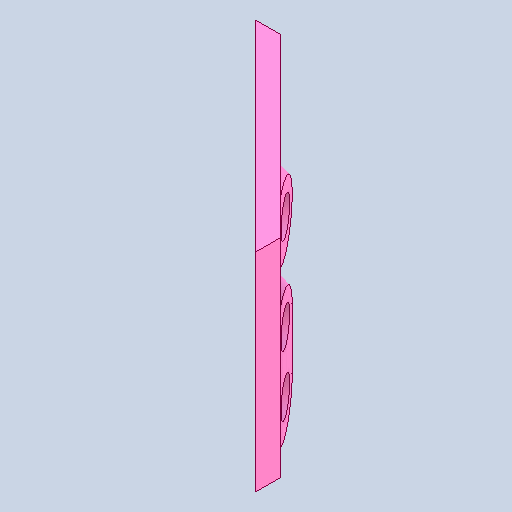
# Autodesk Inventor part: Mirror Plate
Saved by Autodesk Inventor 2023.1 (Build 271208000, 208)
## iProperties
Created: 2022-08-09
Part Number: Mirror Plate
Material: Generic
Document SubType Name: Modeling
Designer: xSibe
Density: 1 g/cm^3
Appearance: Plastic Pink
Author: xSibe
Autodesk Inventor part; units mm, degrees
ref_plane "YZ Plane" through (0, 0, 0) normal (1, 0, 0) x (0, 1, 0)
ref_plane "Work Plane1" through (-24.9, -24.9, 7.7) normal (0, 0, 1) x (1, 0, 0)
sketch "Sketch1" plane through (0, 0, 0) normal (0, 0, 1) x (0, 1, 0)
  circle A0 centre (20.9, 10) radius 1.875 projected
  circle A1 centre (-20.9, 10) radius 1.875 projected
  circle A2 centre (20.9, -10) radius 1.875 projected
  circle A3 centre (-20.9, -10) radius 1.875 projected
  circle A4 centre (-14.4, -20.8) radius 2.0675 projected
  circle A5 centre (14.4, -20.8) radius 2.0675 projected
  circle A6 centre (14.4, 20.8) radius 2.0675 projected
  circle A7 centre (-14.4, 20.8) radius 2.0675 projected
  line L0 (-16.9, -16.9) -> (-16.9, 16.9) projected
  line L1 (-16.9, 16.9) -> (16.9, 16.9) projected
  line L2 (16.9, 16.9) -> (16.9, -16.9) projected
  line L3 (16.9, -16.9) -> (-16.9, -16.9) projected
  line L4 (24.9, 17.05) -> (22.55, 17.05) projected
  line L5 (22.55, 17.05) -> (17.05, 22.55) projected
  line L6 (17.05, 22.55) -> (17.05, 24.9) projected
  line L7 (17.05, 24.9) -> (-17.05, 24.9) projected
  line L8 (-17.05, 24.9) -> (-17.05, 22.55) projected
  line L9 (-17.05, 22.55) -> (-22.55, 17.05) projected
  line L10 (-22.55, 17.05) -> (-24.9, 17.05) projected
  line L11 (-24.9, 17.05) -> (-24.9, -17.05) projected
  line L12 (-24.9, -17.05) -> (-22.55, -17.05) projected
  line L13 (-22.55, -17.05) -> (-17.05, -22.55) projected
  line L14 (-17.05, -22.55) -> (-17.05, -24.9) projected
  line L15 (-17.05, -24.9) -> (17.05, -24.9) projected
  line L16 (17.05, -24.9) -> (17.05, -22.55) projected
  line L17 (17.05, -22.55) -> (22.55, -17.05) projected
  line L18 (22.55, -17.05) -> (24.9, -17.05) projected
  line L19 (24.9, -17.05) -> (24.9, 17.05) projected
  line L20 (16.975, -24.825) -> (-16.975, -24.825)
  line L21 (-16.975, -24.825) -> (-16.975, -22.5189)
  line L22 (-16.975, -22.5189) -> (-22.5189, -16.975)
  line L23 (-22.5189, -16.975) -> (-24.825, -16.975)
  line L24 (-24.825, -16.975) -> (-24.825, 16.975)
  line L25 (-24.825, 16.975) -> (-22.5189, 16.975)
  line L26 (-22.5189, 16.975) -> (-16.975, 22.5189)
  line L27 (-16.975, 22.5189) -> (-16.975, 24.825)
  line L28 (-16.975, 24.825) -> (16.975, 24.825)
  line L29 (16.975, 24.825) -> (16.975, 22.5189)
  line L30 (16.975, 22.5189) -> (22.5189, 16.975)
  line L31 (22.5189, 16.975) -> (24.825, 16.975)
  line L32 (24.825, 16.975) -> (24.825, -16.975)
  line L33 (24.825, -16.975) -> (22.5189, -16.975)
  line L34 (22.5189, -16.975) -> (16.975, -22.5189)
  line L35 (16.975, -22.5189) -> (16.975, -24.825)
  dimension "d5" = 0.075
  constraints: 32 end point, 15 other
  measures "d5" distance between parallel lines of L15 L20
extrude "Extrusion1" add sketch "Sketch1" along normal blind 2.5 from surface at 7.7 contours A0 | A1 | A2 | A3 | A4 | A5 | A6 | A7 | L0 L1 L2 L3 | L20 L21 L22 L23 L24 L25 L26 L27 L28 L29 L30 L31 L32 L33 L34 L35
sketch "Sketch2" plane through (0, 0, 0) normal (0, 1, 0) x (-1, 0, 0)
  line L0 (16.975, 10.2) -> (-16.975, 10.2) projected
  line L1 (-16.975, 7.7) -> (-16.975, 10.2) projected
  line L2 (16.975, 7.7) -> (-16.975, 7.7) projected
  line L3 (16.975, 7.7) -> (16.975, 10.2) projected
  line L4 (16.975, 7.7) -> (-16.975, 41.65)
  line L5 (16.975, 7.7) -> (64.9876, 7.7) construction
  line L6 (-16.975, 41.65) -> (-16.975, 10.2)
  line L7 (-20.5105, 41.65) -> (10.9395, 10.2)
  line L8 (7.4039, 10.2) -> (-24.0461, 41.65)
  line L9 (-19.475, 12.7) -> (19.475, 12.7)
  line L10 (19.475, 12.7) -> (19.475, 5.2)
  line L11 (19.475, 5.2) -> (-19.475, 5.2)
  line L12 (-19.475, 5.2) -> (-19.475, 12.7)
  line L13 (-16.975, 41.65) -> (-24.825, 41.65)
  line L14 (-24.825, 41.65) -> (-24.825, 10.2)
  line L15 (-24.825, 10.2) -> (-16.975, 10.2)
  line L16 (-16.975, 10.2) -> (-16.975, 41.65)
  point P0 (0, 0)
  point P1 (14.475, 10.2)
  point P2 (-16.975, 38.1145)
  point P3 (-16.975, 34.5789)
  point P4 (8.4395, 12.7)
  point P5 (11.975, 12.7)
  point P6 (-19.475, 10.2)
  point P7 (-16.975, 12.7)
  point P8 (-16.975, 10.2)
  dimension "d6" = 135
  dimension "d9" = 2.5
  dimension "d10" = 2.5
  dimension "d13" = 2.5
  constraints: 26 end point, 8 point on line, 2 horizontal, 2 parallel, 2 perpendicular, 1 equal length, 3 other
  measures "d6" angle of L5 L4
  measures "d9" distance between parallel lines of L4 L7
  measures "d10" distance between parallel lines of L7 L8
  measures "d13" distance between parallel lines of L0 L9
extrude "Extrusion2" add sketch "Sketch2" along normal mid plane 30 contours L7 L9 L4 L0 | L0 L8 L9 L7 | L0 L6 L9 L8 | L9 L8 L6 L7 | L7 L6 L4 L9 | L15 L12 L9 L6 | L9 L6 L8 | L7 L13 L6 | L6 L8 L13 L7 | L9 L12 L15 L14 L13 L8 L6
extrude "Extrusion3" cut sketch "Sketch2" along normal mid plane 30 contours L7 L9 L4 L0 | L0 L8 L9 L7 | L9 L8 L6 L7 | L7 L13 L6 | L6 L8 L13 L7
ref_plane "Work Plane2" through (24.825, 0, 41.65) normal (0.9848078, 0, -0.1736482) x (0, 1, 0)
sketch "Sketch3" plane through (20.7643, -15, 18.6207) normal (0.9848078, 0, -0.1736482) x (-0.1736482, 0, -0.9848078)
  line L0 (10.902, 0) -> (-18.5396, 0) projected
  line L1 (10.902, 0) -> (10.902, 30) projected
  line L2 (-18.5396, 30) -> (10.902, 30) projected
  line L3 (-18.5396, 15) -> (10.902, 15)
  line L4 (6.1812, 6.25) -> (-13.8188, 6.25)
  line L5 (-13.8188, 6.25) -> (-13.8188, 23.75)
  line L6 (-13.8188, 23.75) -> (6.1812, 23.75)
  line L7 (6.1812, 23.75) -> (6.1812, 6.25)
  line L8 (6.1812, 6.25) -> (-13.8188, 23.75) construction
  line L9 (-13.8188, 6.25) -> (6.1812, 23.75) construction
  circle A0 centre (-13.8188, 6.25) radius 2.5875
  circle A1 centre (-13.8188, 6.25) radius 5.0875
  line L10 (-3.8188, 15) -> (-3.8188, 6.25)
  line L11 (-3.8188, 10.625) -> (-13.8188, 10.625)
  line L12 (-8.8188, 10.625) -> (-8.8188, 6.25)
  circle A2 centre (-13.8188, 15) radius 2.5875
  circle A3 centre (-13.8188, 15) radius 5.0875
  circle A4 centre (-3.8188, 15) radius 5.0875
  circle A5 centre (-3.8188, 15) radius 2.5875
  line L13 (-18.9063, 6.25) -> (-18.9063, 15)
  line L14 (-8.7313, 15) -> (-8.7313, 6.25)
  line L15 (-18.5396, 0) -> (-18.5396, 30) projected
  point P0 (21.9435, 15)
  dimension "d16" = 20
  dimension "d17" = 17.5
  dimension "d18" = 5.175
  dimension "d19" = 2.5
  constraints: 24 end point, 8 midpoint, 6 centre point, 5 point on line, 4 point on circle, 3 perpendicular, 2 parallel, 1 coincident, 1 horizontal, 1 symmetric about line, 1 tangent, 4 other
  measures "d16" distance of L5.end L6.end
  measures "d17" distance of L4.end L5.end
  measures "d18" diameter of A0
  measures "d19" radial gap between concentric circles of A0 A1
extrude "Extrusion4" cut sketch "Sketch3" along normal mid plane 50 contours A0 L5 L4 | L4 L5 A0 | A2 L3 L5 | L5 L3 A2 | A2 L5 L3 | A2 L3 L5
extrude "Extrusion5" cut sketch "Sketch3" along normal blind 4.25 and the other way blind 2.5 contours L15 A1 A3 L5 A0 L4 | A1 L15 | L13 A3 L15 A1 | L4 L12 A1 | A1 L12 L11 L14 | L15 A3 A1 | A3 L15 | L4 A0 L5 A3 A1 L12 | A1 L11 L12 | L11 A3 A4 L14 | A3 L15 L3 A2 L5 A1 | A1 L5 A3 | A3 L5 A2 L3 L15 | A4 L3 A2 L5 A3 | A3 L3 A4 | A0 L5 L4 | L4 L5 A0 | L11 L5 A1 | A3 L5 L11 | A1 L5 A2 L3 A4 A3 | A4 A3 L14 | A3 A4 L3 | A2 L3 L5 | L5 L3 A2 | A2 L5 L3 | A2 L3 L5
sketch "Sketch4" plane through (17.8921, 0, 2.3313) normal (0.9848078, 0, -0.1736482) x (0, 1, 0)
  line L0 (-15, 5.6387) -> (-15, 35.0803) projected
  line L1 (-15, 5.6387) -> (15, 5.6387) projected
  line L2 (15, 35.0803) -> (15, 5.6387) projected
  circle A0 centre (0, 14.3887) radius 2.5875
  circle A1 centre (0, 14.3887) radius 5.0875
  line L3 (-15, 35.0803) -> (15, 35.0803) projected
  line L4 (0, 5.6387) -> (0, 14.3887)
  point P0 (0, -5.1645)
  dimension "d25" = 5.175
  dimension "d26" = 2.5
  dimension "d37" = 8.75
  constraints: 2 centre point, 2 end point, 1 coincident, 1 midpoint, 1 vertical
  measures "d25" diameter of A0
  measures "d26" radial gap between concentric circles of A0 A1
  measures "d37" distance of L4.start L4.end
extrude "Extrusion6" cut sketch "Sketch4" along normal mid plane 100 contours A0
extrude "Extrusion7" cut sketch "Sketch4" along normal blind 15 and the other way blind 10 contours A0 | A1
sketch "Sketch7" plane through (-3.5875, 0, 17.552) normal (0, 1, 0) x (-0.7071068, 0, -0.7071068)
  line L0 (-20.158, 0) -> (-26.4755, 0) projected
  line L1 (-0.6613, 0) -> (-6.9788, 0) projected
  line L2 (1.0892, 2.5) -> (-0.6613, 0) projected
  line L3 (-5.2283, 2.5) -> (1.0892, 2.5) projected
  line L4 (-5.2283, 2.5) -> (-6.9788, 0) projected
  line L5 (-18.4075, 2.5) -> (-20.158, 0) projected
  line L6 (-24.725, 2.5) -> (-18.4075, 2.5) projected
  line L7 (-24.725, 2.5) -> (-26.4755, 0) projected
  line L8 (-3.8201, 0) -> (-4.0701, 0)
  line L9 (-23.3168, 0) -> (-23.5668, 0)
  line L10 (-1.7448, -1.4254) -> (-6.7427, -0.5442)
  line L11 (-6.7427, -0.5442) -> (-6.3954, 1.4254)
  line L12 (-6.3954, 1.4254) -> (-1.3975, 0.5442)
  line L13 (-1.3975, 0.5442) -> (-1.7448, -1.4254)
  line L14 (-1.7448, -1.4254) -> (-6.3954, 1.4254) construction
  line L15 (-6.7427, -0.5442) -> (-1.3975, 0.5442) construction
  line L16 (-1.7448, -1.4254) -> (3.3302, -1.4254) construction
  line L17 (-21.2415, -1.4254) -> (-26.2394, -0.5442)
  line L18 (-26.2394, -0.5442) -> (-25.8921, 1.4254)
  line L19 (-25.8921, 1.4254) -> (-20.8942, 0.5442)
  line L20 (-20.8942, 0.5442) -> (-21.2415, -1.4254)
  line L21 (-21.2415, -1.4254) -> (-25.8921, 1.4254) construction
  line L22 (-26.2394, -0.5442) -> (-20.8942, 0.5442) construction
  line L23 (-21.2415, -1.4254) -> (-16.1665, -1.4254) construction
  line L24 (-27.1088, 3.1631) -> (-27.9771, -1.7609)
  line L25 (-27.9771, -1.7609) -> (-20.0247, -3.1631)
  line L26 (-20.0247, -3.1631) -> (-19.1565, 1.7609)
  line L27 (-19.1565, 1.7609) -> (-27.1088, 3.1631)
  line L28 (-7.6121, 3.1631) -> (-8.4804, -1.7609)
  line L29 (-8.4804, -1.7609) -> (-0.528, -3.1631)
  line L30 (-0.528, -3.1631) -> (0.3402, 1.7609)
  line L31 (0.3402, 1.7609) -> (-7.6121, 3.1631)
  line L32 (-0.6613, 0) -> (0.0297, 0)
  line L33 (-20.158, 0) -> (-19.467, 0)
  line L34 (-1.7448, -1.4254) -> (0.0297, 0)
  line L35 (-21.2415, -1.4254) -> (-19.467, 0)
  line L36 (-26.4755, 0) -> (-27.6666, 0)
  line L37 (-6.9788, 0) -> (-8.1699, 0)
  line L38 (-6.7427, -0.5442) -> (-8.1699, 0)
  line L39 (-26.2394, -0.5442) -> (-27.6666, 0)
  point P0 (-1.4934, 0)
  point P1 (-6.6467, 0)
  point P2 (-26.1434, 0)
  point P3 (-20.9901, 0)
  dimension "d70" = 0.25
  dimension "d71" = 0.25
  dimension "d72" = 5.075
  dimension "d73" = 170
  dimension "d74" = 2
  dimension "d75" = 5.075
  dimension "d76" = 170
  dimension "d77" = 2
  dimension "d78" = 1.5
  dimension "d79" = 1.5
  constraints: 64 end point, 8 parallel, 8 point on line, 6 midpoint, 5 perpendicular, 4 horizontal, 2 equal length, 6 other
  measures "d70" distance of L8.start L8.end
  measures "d71" distance of L9.start L9.end
  measures "d72" distance of L10.start L10.end
  measures "d73" angle of L16 L10
  measures "d74" distance of L10.end L11.end
  measures "d75" distance of L17.start L17.end
  measures "d76" angle of L23 L17
  measures "d77" distance of L17.end L18.end
  measures "d78" distance between parallel lines of L18 L24
  measures "d79" distance between parallel lines of L11 L28
extrude "Extrusion10" add sketch "Sketch7" along normal mid plane 30 contours L0 L18 L7 L19 L20 | L20 L19 L7 L6 L27 L26 L5 L0 | L0 L7 L18 | L26 L27 L6 L5 | L1 L11 L4 L12 L13 | L13 L12 L4 L3 L31 L30 L2 L1 | L1 L4 L11 | L30 L31 L3 L2
extrude "Extrusion11" cut sketch "Sketch7" along normal mid plane 5.075 contours L0 L20 L17 L18 | L0 L18 L7 L19 L20 | L18 L19 L7 | L1 L13 L10 L11 | L1 L11 L4 L12 L13 | L11 L12 L4
sketch "Sketch8" plane through (13.713, -15.0375, 36.8684) normal (0.819152, 0, -0.5735764) x (-0.5735764, 0, -0.819152)
  line L0 (0, 12.5) -> (0, 17.575) projected
  line L1 (5.075, 17.575) -> (5.075, 12.5) projected
  line L2 (0, 12.5) -> (5.075, 12.5) projected
  line L3 (5.075, 17.575) -> (0, 17.575) projected
  line L4 (2.5375, 12.5) -> (2.5375, 17.575)
  circle A0 centre (2.5375, 15.0375) radius 2.5375
  circle A1 centre (2.5375, 15.0375) radius 4.0375
  circle A2 centre (2.5375, 6.2875) radius 4.0375
  circle A3 centre (2.5375, 6.2875) radius 2.5375
  line L5 (-1.5, 6.2875) -> (-1.5, 15.0375)
  line L6 (6.575, 6.2875) -> (6.575, 15.0375)
  point P0 (38.0663, 15.0375)
  dimension "d86" = 5.075
  dimension "d87" = 1.5
  dimension "d90" = 8.75
  constraints: 6 end point, 4 centre point, 4 point on circle, 4 tangent, 3 midpoint, 1 vertical, 3 other
  measures "d86" diameter of A0
  measures "d87" radial gap between concentric circles of A0 A1
  measures "d90" distance of A0.centre A3.centre
extrude "Extrusion12" cut sketch "Sketch8" along normal blind 1.5 contours A0 L4 | L4 A0 | A3
extrude "Extrusion13" add sketch "Sketch8" along normal blind 1.5 contours L0 A0 L2 | L0 L3 A0 | A0 L1 L2 | L3 L1 A0 | A1 | L6 A2 L5 A1 | A2
sketch "Sketch9" plane through (-0.0732, -2.5375, 23.0821) normal (0.819152, 0, -0.5735764) x (-0.5735764, 0, -0.819152)
  line L0 (0, 0) -> (0, 5.075) projected
  line L1 (0, 0) -> (5.075, 0) projected
  line L2 (5.075, 5.075) -> (5.075, 0) projected
  line L3 (5.075, 5.075) -> (0, 5.075) projected
  line L4 (2.5375, 0) -> (2.5375, 5.075)
  circle A0 centre (2.5375, 2.5375) radius 2.5375
  circle A1 centre (2.5375, 2.5375) radius 4.0375
  point P0 (18.8658, 2.5375)
  dimension "d99" = 5.075
  dimension "d100" = 1.5
  constraints: 3 midpoint, 2 centre point, 2 end point
  measures "d99" diameter of A0
  measures "d100" radial gap between concentric circles of A0 A1
extrude "Extrusion14" add sketch "Sketch9" along normal blind 1.5 contours L0 A0 L1 | L0 L3 A0 | A0 L2 L1 | L3 L2 A0 | A1
chamfer "Chamfer1" distance 1.21 angle 45 3 edges at (11.9583, -12.4749, 33.0978) (-1.8279, 3.7249, 19.3115) (-1.8279, -3.7249, 19.3115)
sketch "Sketch10" plane through (0, 0, 0) normal (0, 1, 0) x (-1, 0, 0)
  line L0 (8.4395, 12.7) -> (-16.975, 38.1145) projected
  line L1 (-16.975, 38.1145) -> (-16.975, 41.65) projected
  line L2 (-16.975, 41.65) -> (11.975, 12.7) projected
  line L3 (11.975, 12.7) -> (8.4395, 12.7) projected
  line L4 (-11.1764, 30.6305) -> (-15.1128, 36.2522) projected
  line L5 (-11.1689, 30.6232) -> (-11.1764, 30.6305) projected
  line L6 (-15.1128, 36.2522) -> (-9.3221, 30.4616) projected
  line L7 (-1.3265, 22.466) -> (2.6099, 16.8443) projected
  line L8 (2.6099, 16.8443) -> (2.6099, 16.8443) projected
  line L9 (2.6099, 16.8443) -> (-1.3265, 22.466) projected
  line L10 (-1.3265, 22.466) -> (-1.3265, 22.466) projected
  line L11 (-24.0461, 41.65) -> (7.4039, 10.2) projected
  line L12 (-24.825, 10.2) -> (7.4039, 10.2) projected
  line L13 (-24.825, 10.2) -> (-24.825, 41.65) projected
  line L14 (-24.825, 41.65) -> (-24.0461, 41.65) projected
  line L15 (22.5189, 10.2) -> (24.825, 10.2) projected
  line L16 (24.825, 7.7) -> (24.825, 10.2) projected
  line L17 (22.5189, 7.7) -> (24.825, 7.7) projected
  line L18 (22.5189, 7.7) -> (22.5189, 10.2) projected
  line L19 (16.975, 10.2) -> (22.5189, 10.2) projected
  line L20 (22.5189, 7.7) -> (22.5189, 10.2) projected
  line L21 (16.975, 7.7) -> (22.5189, 7.7) projected
  line L22 (16.975, 7.7) -> (16.975, 10.2) projected
  line L23 (-16.975, 10.2) -> (16.975, 10.2) projected
  line L24 (16.975, 7.7) -> (16.975, 10.2) projected
  line L25 (-16.975, 7.7) -> (16.975, 7.7) projected
  line L26 (-16.975, 7.7) -> (-16.975, 10.2) projected
  line L27 (-22.5189, 10.2) -> (-16.975, 10.2) projected
  line L28 (-16.975, 7.7) -> (-16.975, 10.2) projected
  line L29 (-22.5189, 7.7) -> (-16.975, 7.7) projected
  line L30 (-22.5189, 7.7) -> (-22.5189, 10.2) projected
  line L31 (-24.825, 10.2) -> (-22.5189, 10.2) projected
  line L32 (-22.5189, 7.7) -> (-22.5189, 10.2) projected
  line L33 (-24.825, 7.7) -> (-22.5189, 7.7) projected
  line L34 (-24.825, 7.7) -> (-24.825, 10.2) projected
  line L35 (2.6099, 16.8443) -> (8.4395, 12.7)
  line L36 (-11.1764, 30.6305) -> (-1.3265, 22.466)
  line L37 (-11.1689, 30.6232) -> (-9.3221, 30.4616) projected
  point P0 (0, 0)
  constraints: 4 end point
extrude "Extrusion15" cut sketch "Sketch10" along normal mid plane 50 contours L11 L12 L13 L14 | L23 L22 L25 L26 L12 | L26 L29 L30 L12 | L19 L18 L21 L22 | L12 L30 L33 L34 | L15 L16 L17 L18
body "Solid1"
